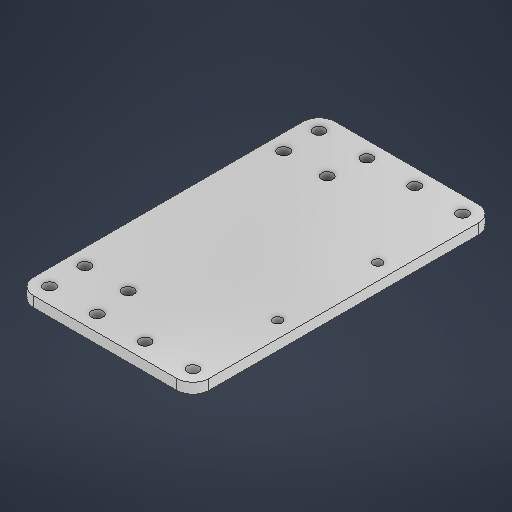
# Autodesk Inventor part: CNC-016-SpindleMountPlate
Saved by Autodesk Inventor 2026.2 (Build 302298000, 298)
## iProperties
Created: 2026-06-20
Part Number: CNC-016-SpindleMountPlate
Material: Aluminum 6061
Document SubType Name: Modeling
Designer: Kenji
Density: 2.7 g/cm^3
Appearance: Aluminum - Dark
Author: Kenji
Autodesk Inventor part; units mm, degrees
ref_plane "YZ Plane" through (0, 0, 0) normal (1, 0, 0) x (0, 1, 0)
ref_plane "XZ Plane" through (0, 0, 0) normal (0, 1, 0) x (-1, 0, 0)
ref_plane "XY Plane" through (0, 0, 0) normal (0, 0, 1) x (1, 0, 0)
sketch "Sketch1" plane through (0, 0, 0) normal (0, 1, 0) x (-1, 0, 0)
  circle A0 centre (0, 0) radius 2.1
  circle A1 centre (0, 46) radius 2.1
  circle A2 centre (0, -39) radius 2.6
  circle A3 centre (66, -39) radius 2.6
  circle A4 centre (46, -22.7383) radius 2.6
  circle A5 centre (66, -22.7383) radius 2.6
  circle A6 centre (44, -39) radius 2.6
  circle A7 centre (22, -39) radius 2.6
  line L0 (0, 23) -> (66, 23) construction
  circle A8 centre (0, 85) radius 2.6
  circle A9 centre (66, 85) radius 2.6
  circle A10 centre (46, 68.7383) radius 2.6
  circle A11 centre (66, 68.7383) radius 2.6
  circle A12 centre (44, 85) radius 2.6
  circle A13 centre (22, 85) radius 2.6
  circle A14 centre (66, -39) radius 7.3625 construction
  circle A15 centre (66, 85) radius 7.3625 construction
  circle A16 centre (0, 85) radius 7.3625 construction
  circle A17 centre (0, -39) radius 7.3625 construction
  line L1 (73.3625, -39) -> (73.3625, 85)
  line L2 (66, -46.3625) -> (0, -46.3625)
  line L3 (-7.3625, -39) -> (-7.3625, 85)
  line L4 (0, 92.3625) -> (66, 92.3625)
  arc A18 (66, -46.3625) -> (73.3625, -39) centre (66, -39) ccw
  arc A19 (-7.3625, -39) -> (0, -46.3625) centre (0, -39) ccw
  arc A20 (0, 92.3625) -> (-7.3625, 85) centre (0, 85) ccw
  arc A21 (73.3625, 85) -> (66, 92.3625) centre (66, 85) ccw
  dimension "d0" = 4.2
  dimension "d1" = 46
  dimension "d2" = 39
  dimension "d3" = 66
  dimension "d4" = 20
  dimension "d6" = 22
  dimension "d7" = 22
  dimension "d8" = 23
  dimension "d9" = 4.7625
  dimension "d12" = 91.4766
  dimension "d13" = 5.2
  constraints: 22 centre point, 16 point on circle, 13 equal radius, 10 end point, 7 tangent, 6 symmetric about line, 5 vertical alignment, 4 coincident, 4 horizontal alignment, 1 horizontal, 1 perpendicular, 6 other
  measures "d0" diameter of A0
  measures "d1" distance of point (0, 0) A1.centre
  measures "d2" distance of A2.centre point (0, 0)
  measures "d3" distance of A3.centre A2.centre
  measures "d4" distance of A4.centre A5.centre
  measures "d6" distance of A2.centre A7.centre
  measures "d7" distance of A7.centre A6.centre
  measures "d8" distance from line of L0 A1.centre
  measures "d9" radial gap between concentric circles of A14 A3
  measures "d12" distance of A10.centre A4.centre
  measures "d13" diameter of A2
extrude "Extrusion1" add sketch "Sketch1" along normal blind 4.7625
equation "\"d6\" = 0.333333 * d3"
equation "\"d7\" = d6"
equation "\"d8\" = 0.5 * d1"
body "Solid1"
